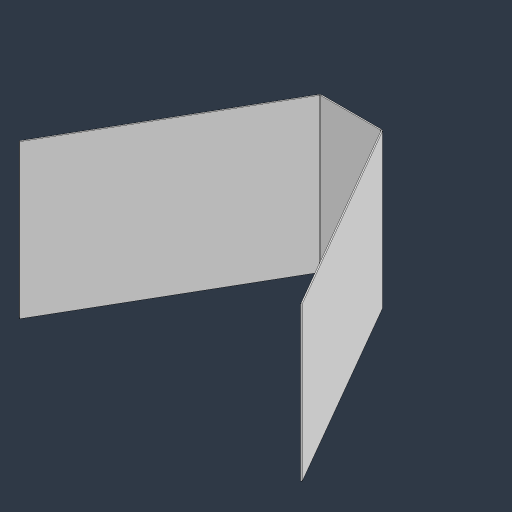
# Autodesk Inventor part: hopper
Saved by Autodesk Inventor 2024.3 (Build 283343000, 343)
## iProperties
Created: 2025-03-05
Part Number: hopper
Material: Generic
Document SubType Name: Sheet Metal
Designer: Marcus Tannini
Density: 1 g/cm^3
Sheet Metal Rule: Default
Appearance: Default
Author: Marcus Tannini
Autodesk Inventor part; units mm, degrees
ref_plane "YZ Plane" through (0, 0, 0) normal (1, 0, 0) x (0, 1, 0)
ref_plane "XZ Plane" through (0, 0, 0) normal (0, 1, 0) x (-1, 0, 0)
ref_plane "XY Plane" through (0, 0, 0) normal (0, 0, 1) x (1, 0, 0)
sketch "Sketch1" plane through (0, 0, 0) normal (0, 0, 1) x (1, 0, 0)
  line L0 (-82.55, -203.2) -> (82.55, -203.2)
  line L1 (82.55, -203.2) -> (82.55, 203.2)
  line L2 (82.55, 203.2) -> (-82.55, 203.2)
  line L3 (-82.55, 203.2) -> (-82.55, -203.2)
  line L4 (-82.55, -203.2) -> (82.55, 203.2) construction
  line L5 (82.55, -203.2) -> (-82.55, 203.2) construction
  point P0 (0, 0)
  dimension "d0" = 165.1
  dimension "d1" = 406.4
  measures "d0" distance of L2.end L1.end
  measures "d1" distance of L0.end L1.end
extrude "Plate1" add sketch "Sketch1" along normal blind 3.048
sketch "Sketch2" plane through (79.9104, 203.2, 1.524) normal (0.8660254, 0, -0.5) x (0, 1, 0)
  line L0 (-406.4, 0) -> (0, 0)
  line L1 (0, 0) -> (0, 584.2)
  line L2 (0, 584.2) -> (-406.4, 584.2)
  line L3 (-406.4, 584.2) -> (-406.4, 0)
  constraints: 6 end point, 1 horizontal, 1 perpendicular, 1 vertical
edge flange "Flange1" height 584.2 angle 60 thickness 3.048 bend radius 3.048 thickness toward (0.8660254, 0, -0.5) relief straight relief width 3.048 relief depth 1.524 corner gap 3.048 corner form 0 edges at (82.55, 0, 3.048) (-82.55, 0, 3.048) wall of the first edge with corners at (79.9104, -203.2, 1.524) (79.9104, 203.2, 1.524) (372.0104, 203.2, 507.456) (372.0104, -203.2, 507.456)
bend "Bend1"
corner "Corner1"
equation "\"d2\" = Thickness"
equation "\"d3\" = BendReliefWidth"
equation "\"d4\" = BendReliefDepth"
equation "\"d5\" = MinimumRemnant"
equation "\"d6\" = TransitionRadius"
equation "\"d9\" = BendRadius"
equation "\"d10\" = CornerReliefSize"
equation "\"d11\" = GapSize"
equation "\"d12\" = JacobiRadiusSize"
equation "\"BendRadius\" = Thickness"
equation "\"BendReliefWidth\" = Thickness"
equation "\"BendReliefDepth\" = 0.5 * Thickness"
equation "\"CornerReliefSize\" = 4 * Thickness"
equation "\"MinimumRemnant\" = 2 * Thickness"
equation "\"TransitionRadius\" = BendRadius"
equation "\"JacobiRadiusSize\" = BendRadius"
equation "\"GapSize\" = Thickness"
equation "\"Thickness\" = 3.048"
body "Solid1"
